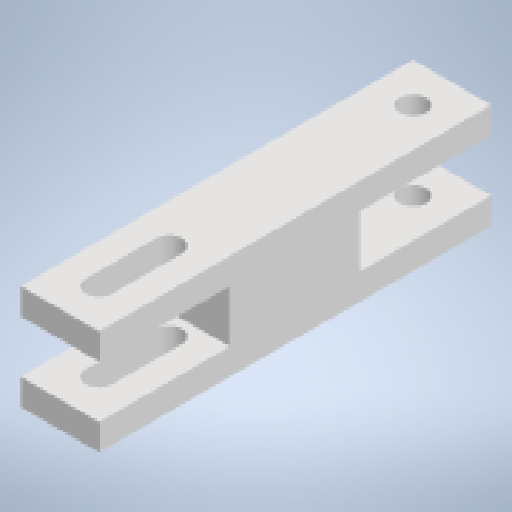
# Autodesk Inventor part: intermig_2
Saved by Autodesk Inventor 2024.3 (Build 283343000, 343)
## iProperties
Created: 2024-05-13
Part Number: intermig_2
Material: Genérico
Document SubType Name: Modeling
Designer: riera
Density: 1 g/cm^3
Appearance: Valor por defecto
Author: riera
Autodesk Inventor part; units mm, degrees
ref_plane "YZ Plane" through (0, 0, 0) normal (1, 0, 0) x (0, 1, 0)
ref_plane "XZ Plane" through (0, 0, 0) normal (0, 1, 0) x (-1, 0, 0)
ref_plane "XY Plane" through (0, 0, 0) normal (0, 0, 1) x (1, 0, 0)
sketch "Boceto1" plane through (0, 0, 0) normal (0, 0, 1) x (1, 0, 0)
  line L0 (-4.5, 6) -> (4.5, 6)
  line L1 (4.5, 6) -> (4.5, -6)
  line L2 (4.5, -6) -> (-4.5, -6)
  line L3 (-4.5, -6) -> (-4.5, 6)
  point P0 (0, 0)
  point P1 (0, 6)
  point P2 (4.5, 0)
  dimension "d0" = 9
  dimension "d1" = 12
  constraints: 8 end point, 2 midpoint, 2 parallel, 1 horizontal, 1 horizontal alignment, 1 perpendicular, 1 vertical alignment
  measures "d0" distance of L0.start L0.end
  measures "d1" distance of L0.end L1.end
extrude "Extrusión1" add sketch "Boceto1" along normal blind 45
sketch "Boceto2" plane through (0, 0, 0) normal (0, 0, -1) x (-1, 0, 0)
  line L0 (4.5, -3) -> (-4.5, -3)
  line L1 (-4.5, -3) -> (-4.5, 3)
  line L2 (-4.5, 3) -> (4.5, 3)
  line L3 (4.5, 3) -> (4.5, -3)
  line L4 (4.5, 6) -> (4.5, -6) projected
  point P0 (0, 0)
  point P1 (-4.5, 0)
  point P2 (0, -3)
  dimension "d4" = 6
  constraints: 8 end point, 2 midpoint, 2 parallel, 1 collinear, 1 horizontal, 1 horizontal alignment, 1 perpendicular, 1 vertical alignment
  measures "d4" distance of L2.end L0.start
extrude "Extrusión2" cut sketch "Boceto2" against normal blind 15
ref_plane "Plano de trabajo1" through (0, 0, 22.5) normal (0, 0, 1) x (1, 0, 0)
sketch "Boceto3" plane through (-4.5, -6, 0) normal (0, -1, 0) x (1, 0, 0)
  circle A0 centre (4.5, 4.5) radius 1.5
  line L0 (0, 0) -> (9, 0) projected
  point P0 (4.5, 0)
  point P1 (4.5, 0)
  point P2 (4.5, 0)
  dimension "d8" = 3
  dimension "d9" = 4.5
  constraints: 2 midpoint, 1 centre point, 1 vertical alignment
  measures "d8" diameter of A0
  measures "d9" distance of point (4.5, 0) A0.centre
extrude "Extrusión3" cut sketch "Boceto3" against normal through all
mirror "Simetría2" about plane through (0, 0, 22.5) normal (0, 0, 1) of "Extrusión2"
sketch "Boceto4" plane through (-4.5, 6, 0) normal (0, 1, 0) x (1, 0, 0)
  line L0 (3, -32.5) -> (3, -40.5)
  line L1 (6, -40.5) -> (6, -32.5)
  line L2 (9, 0) -> (9, -45) projected
  line L3 (9, -45) -> (0, -45) projected
  arc A0 (6, -32.5) -> (3, -32.5) centre (4.5, -32.5) ccw
  arc A1 (3, -40.5) -> (6, -40.5) centre (4.5, -40.5) ccw
  line L4 (9, -30) -> (0, -30) projected
  point P0 (4.5, 0)
  dimension "d13" = 3
  dimension "d15" = 8
  dimension "d16" = 4.5
  dimension "d17" = 1.5
  constraints: 4 end point, 4 point on circle, 4 tangent, 2 centre point, 1 parallel
  measures "d13" distance between parallel lines of L2 L1
  measures "d15" distance of A0.centre A1.centre
  measures "d16" distance from line of L3 A1.centre
  measures "d17" radius of A0
extrude "Extrusión4" cut sketch "Boceto4" against normal through all
scale "Escala1" factors (0.8, 0.8, 0.8) then translate (0, 1.2, 4.5) bodies 1
